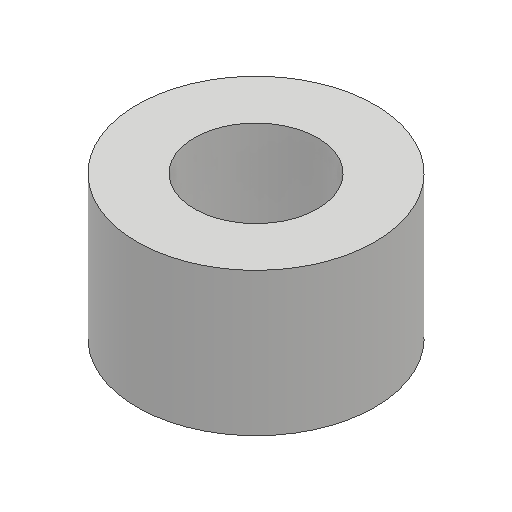
# Autodesk Inventor part: 3DP_ABS_Chamber_Fan_Cover_Spacer
Saved by Autodesk Inventor 2026.1 (Build 301233000, 233)
## iProperties
Created: 2017-07-28
Part Number: 3DP_ABS_Chamber_Fan_Cover_Spacer
Material: Ogólny
Document SubType Name: Modeling
Designer: Andrzej
Density: 1 g/cm^3
Appearance: Domyślna
Author: Andrzej
Autodesk Inventor part; units mm, degrees
ref_plane "YZ Plane" through (0, 0, 0) normal (1, 0, 0) x (0, 1, 0)
ref_plane "XZ Plane" through (0, 0, 0) normal (0, 1, 0) x (-1, 0, 0)
ref_plane "XY Plane" through (0, 0, 0) normal (0, 0, 1) x (1, 0, 0)
sketch "Szkic1" plane through (0, 0, 0) normal (0, 0, 1) x (1, 0, 0)
  circle A0 centre (0, 0) radius 2.15
  circle A1 centre (0, 0) radius 4.15
  dimension "d0" = 4.3
  dimension "d1" = 2
  constraints: 2 centre point, 1 coincident
  measures "d0" diameter of A0
  measures "d1" radial gap between concentric circles of A0 A1
extrude "Wyciągnięcie proste1" add sketch "Szkic1" along normal blind 5
